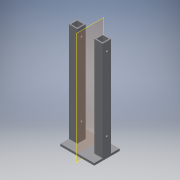
# Autodesk Inventor part: catapultArmSupportStructure
Saved by Autodesk Inventor 2016 SP1 (Build 200210100, 210)
## iProperties
Created: 2016-01-12
Part Number: catapultArmSupportStructure
Material: Generic
Document SubType Name: Modeling
Designer: steele
Density: 1 g/cm^3
Appearance: Default
Author: steele
Autodesk Inventor part; units mm, degrees
ref_plane "XZ Plane" through (0, 0, 0) normal (0, 1, 0) x (-1, 0, 0)
ref_plane "XY Plane" through (0, 0, 0) normal (0, 0, 1) x (1, 0, 0)
sketch "Sketch4" plane through (0, 0, 0) normal (0, 1, 0) x (-1, 0, 0)
  line L0 (-50.8, 38.1) -> (-50.8, -38.1)
  line L1 (-50.8, -38.1) -> (50.8, -38.1)
  line L2 (50.8, -38.1) -> (50.8, 38.1)
  line L3 (50.8, 38.1) -> (-50.8, 38.1)
  line L4 (-50.8, 38.1) -> (50.8, -38.1) construction
  line L5 (-50.8, -38.1) -> (50.8, 38.1) construction
  point P0 (0, 0)
  dimension "d14" = 76.2
  dimension "d15" = 101.6
  constraints: 12 end point, 2 midpoint, 2 parallel, 1 perpendicular, 1 vertical
  measures "d14" distance of L0.start L0.end
  measures "d15" distance of L2.end L0.start
extrude "Extrusion4" add sketch "Sketch4" along normal blind 6.35
sketch "Sketch6" plane through (0, 6.35, 0) normal (0, 1, 0) x (1, 0, 0)
  line L0 (-50.8, 38.1) -> (-50.8, -38.1) construction
  line L1 (-50.8, 0) -> (50.8, 0) construction
  line L2 (50.8, -38.1) -> (50.8, 38.1) construction
  line L3 (-50.8, -12.7) -> (-25.4, -12.7)
  line L4 (-25.4, -12.7) -> (-25.4, 12.7)
  line L5 (-25.4, 12.7) -> (-50.8, 12.7)
  line L6 (-50.8, 12.7) -> (-50.8, -12.7)
  line L7 (-50.8, -12.7) -> (-25.4, 12.7) construction
  line L8 (-25.4, -12.7) -> (-50.8, 12.7) construction
  line L9 (-47.625, -9.525) -> (-28.575, -9.525)
  line L10 (-28.575, -9.525) -> (-28.575, 9.525)
  line L11 (-28.575, 9.525) -> (-47.625, 9.525)
  line L12 (-47.625, 9.525) -> (-47.625, -9.525)
  line L13 (-47.625, -9.525) -> (-28.575, 9.525) construction
  line L14 (-28.575, -9.525) -> (-47.625, 9.525) construction
  line L15 (50.8, 38.1) -> (-50.8, 38.1) construction
  line L16 (0, 38.1) -> (0, -38.1) construction
  line L17 (-50.8, -38.1) -> (50.8, -38.1) construction
  line L18 (50.8, -12.7) -> (25.4, -12.7)
  line L19 (25.4, -12.7) -> (25.4, 12.7)
  line L20 (25.4, 12.7) -> (50.8, 12.7)
  line L21 (50.8, 12.7) -> (50.8, -12.7)
  line L22 (47.625, -9.525) -> (28.575, -9.525)
  line L23 (28.575, -9.525) -> (28.575, 9.525)
  line L24 (28.575, 9.525) -> (47.625, 9.525)
  line L25 (47.625, 9.525) -> (47.625, -9.525)
  point P0 (0, 0)
  point P1 (-38.1, 0)
  dimension "d18" = 25.4
  dimension "d19" = 3.175
  constraints: 44 end point, 8 midpoint, 8 symmetric about line, 4 parallel, 4 perpendicular, 1 collinear, 1 point on line
  measures "d18" distance of L5.end L3.start
  measures "d19" distance between parallel lines of L9 L3
extrude "Extrusion5" add sketch "Sketch6" along normal blind 298.45
sketch "Sketch7" plane through (-50.8, 0, -38.1) normal (-1, 0, 0) x (0, 0, 1)
  line L0 (25.4, 304.8) -> (50.8, 304.8) construction
  line L1 (38.1, 304.8) -> (38.1, 0) construction
  point P0 (38.1, 279.4)
  point P1 (38.1, 58.674)
  dimension "d22" = 25.4
  dimension "d24" = 246.126
  constraints: 2 end point, 2 point on line, 1 midpoint, 1 vertical
  measures "d22" distance from line of point (38.1, 279.4) L0
  measures "d24" distance from line of point (38.1, 58.674) L0
hole "Hole1" at (-50.8, 279.4, 0) at (-50.8, 58.674, 0) direction (1, 0, 0) diameter 6.35 end through all
equation "\"d14\" = supportLength"
equation "\"d15\" = supportWidth"
equation "\"d16\" = supportFloorThickness"
equation "\"d18\" = supportTubingSize"
equation "\"d19\" = supportWallTubingThickness"
equation "\"d20\" = supportTubingHeight"
equation "\"d22\" = supportAxelDistanceFromTop"
equation "\"d24\" = supportPulleyAxelDistanceFromTop"
equation "\"d25\" = supportAxelDiam"
equation "\"supportHeight\" = 304.8"
equation "\"supportWidth\" = 101.6"
equation "\"supportLength\" = 76.2"
equation "\"supportSideHoleDiam\" = 6.35"
equation "\"supporttTopWidth\" = 25.4"
equation "\"supportSupportWidth\" = 101.6"
equation "\"supportSupportPullyHeight\" = 127"
equation "\"supportWallTubingThickness\" = 3.175"
equation "\"supportFloorThickness\" = 6.35"
equation "\"supportTubingHeight\" = supportHeight - supportFloorThickness"
equation "\"supportTubingSize\" = 25.4"
equation "\"supportAxelDistanceFromTop\" = 25.4"
equation "\"supportPulleyAxelDistanceFromTop\" = 246.126"
equation "\"supportAxelDiam\" = 6.35"
body "Solid2"
